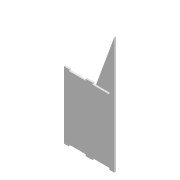
# Autodesk Inventor part: Lateral
Saved by Autodesk Inventor 2022 (Build 260153000, 153)
## iProperties
Created: 2022-06-06
Part Number: Lateral
Material: Generic
Document SubType Name: Modeling
Designer: ADMIN
Density: 1 g/cm^3
Appearance: Default
Author: ADMIN
Autodesk Inventor part; units mm, degrees
ref_plane "YZ Plane" through (0, 0, 0) normal (1, 0, 0) x (0, 1, 0)
ref_plane "XZ Plane" through (0, 0, 0) normal (0, 1, 0) x (-1, 0, 0)
ref_plane "XY Plane" through (0, 0, 0) normal (0, 0, 1) x (1, 0, 0)
sketch "Sketch1" plane through (0, 0, 0) normal (0, 0, 1) x (1, 0, 0)
  line L0 (0, 0) -> (150, 0) projected
  line L1 (150, 0) -> (150, 350) projected
  line L2 (150, 350) -> (95.4045, 200) projected
  line L3 (0, 200) -> (95.4045, 200) projected
  line L4 (0, 0) -> (0, 200) projected
  line L5 (15, 0) -> (65, 0)
  line L6 (65, 0) -> (65, 5)
  line L7 (65, 5) -> (15, 5)
  line L8 (15, 5) -> (15, 0)
  line L9 (85, 0) -> (135, 0)
  line L10 (135, 0) -> (135, 5)
  line L11 (135, 5) -> (85, 5)
  line L12 (85, 5) -> (85, 0)
  line L13 (15, 200) -> (65, 200)
  line L14 (65, 200) -> (65, 195)
  line L15 (65, 195) -> (15, 195)
  line L16 (15, 195) -> (15, 200)
  line L17 (85, 200) -> (135, 200)
  line L18 (135, 200) -> (135, 195)
  line L19 (135, 195) -> (85, 195)
  line L20 (85, 195) -> (85, 200)
  dimension "d0" = 50
  dimension "d1" = 5
  dimension "d2" = 50
  dimension "d3" = 5
  dimension "d4" = 20
  dimension "d5" = 15
  dimension "d6" = 50
  dimension "d7" = 5
  dimension "d8" = 5
  dimension "d9" = 15
  constraints: 32 end point, 8 parallel, 4 horizontal, 4 perpendicular, 4 point on line
  measures "d0" distance of L7.end L6.end
  measures "d1" distance of L6.end L5.end
  measures "d2" distance of L10.end L11.end
  measures "d3" distance of L11.end L9.start
  measures "d4" distance between parallel lines of L12 L6
  measures "d5" distance between parallel lines of L4 L8
  measures "d6" distance of L14.end L15.end
  measures "d7" distance of L13.end L14.end
  measures "d8" distance of L17.end L18.end
  measures "d9" distance between parallel lines of L16 L4
extrude "Extrusion1" add sketch "Sketch1" along normal blind 5 contours L4 L3 L16 L15 L14 L20 L19 L18 L17 L2 L1 L0 L10 L11 L12 L6 L7 L8
sketch "Sketch2" plane through (0, 0, 0) normal (0, 0, -1) x (-1, 0, 0)
  line L0 (-150, 0) -> (-150, 350) projected
  line L1 (-150, 160) -> (-145, 160)
  line L2 (-145, 160) -> (-145, 110)
  line L3 (-145, 110) -> (-150, 110)
  line L4 (-150, 110) -> (-150, 160)
  line L5 (-150, 80) -> (-145, 80)
  line L6 (-145, 80) -> (-145, 30)
  line L7 (-145, 30) -> (-150, 30)
  line L8 (-150, 30) -> (-150, 80)
  line L9 (-135, 0) -> (-150, 0) projected
  point P0 (0, 0)
  dimension "d12" = 5
  dimension "d13" = 50
  dimension "d14" = 5
  dimension "d15" = 50
  dimension "d16" = 30
  dimension "d17" = 30
  constraints: 16 end point, 4 parallel, 2 horizontal, 2 perpendicular, 2 point on line
  measures "d12" distance of L2.end L3.end
  measures "d13" distance of L1.end L2.end
  measures "d14" distance of L6.end L7.end
  measures "d15" distance of L5.end L6.end
  measures "d16" distance between parallel lines of L9 L7
  measures "d17" distance between parallel lines of L3 L5
extrude "Extrusion2" cut sketch "Sketch2" against normal blind 5
equation "\"d2\" = d0"
equation "\"d3\" = d1"
body "Solid1"
